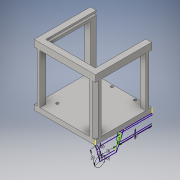
# Autodesk Inventor part: Main_Body_Wheel
Saved by Autodesk Inventor 2016 (Build 200138000, 138)
## iProperties
Created: 2018-09-17
Part Number: Main_Body_Wheel
Material: Generic
Document SubType Name: Modeling
Designer: Kyle
Density: 1 g/cm^3
Appearance: Default
Author: Kyle
Autodesk Inventor part; units mm, degrees
ref_plane "YZ Plane" through (0, 0, 0) normal (1, 0, 0) x (0, 1, 0)
ref_plane "XZ Plane" through (0, 0, 0) normal (0, 1, 0) x (-1, 0, 0)
ref_plane "XY Plane" through (0, 0, 0) normal (0, 0, 1) x (1, 0, 0)
sketch "Sketch1" plane through (0, 0, 0) normal (0, 1, 0) x (-1, 0, 0)
  line L0 (-30, 34) -> (30, 34)
  line L1 (30, 34) -> (30, -34)
  line L2 (30, -34) -> (-30, -34)
  line L3 (-30, -34) -> (-30, 34)
  line L4 (-30, 34) -> (30, -34) construction
  line L5 (30, 34) -> (-30, -34) construction
  line L6 (30, 34) -> (30, 19)
  line L7 (-30, -34) -> (-23, -34)
  line L8 (-30, -34) -> (8.5, -34)
  circle A0 centre (8.5, -31.5) radius 1.5
  circle A1 centre (-19.5, -31.5) radius 1.5
  circle A2 centre (-19.5, -31.5) radius 1.5
  circle A3 centre (24, 19) radius 1.5
  line L9 (24, 19) -> (0, 19)
  line L10 (0, 19) -> (0, 0)
  line L11 (0, 0) -> (8.5, -31.5)
  line L12 (8.5, -31.5) -> (0, -31.5)
  line L13 (-19.5, -31.5) -> (-19.5, 0)
  line L14 (-19.5, 0) -> (0, 0)
  line L15 (30, 34) -> (37, 34)
  line L16 (-37, -34) -> (37, -34)
  line L17 (37, -34) -> (37, 34)
  line L18 (37, 34) -> (-37, 34)
  line L19 (-37, 34) -> (-37, -34)
  line L20 (-37, -34) -> (37, 34) construction
  line L21 (37, -34) -> (-37, 34) construction
  dimension "d0" = 60
  dimension "d1" = 68
  dimension "d3" = 7
  dimension "d5" = 3
  dimension "d6" = 3
  dimension "d7" = 3
  dimension "d10" = 7
  dimension "d11" = 31.5
  dimension "d12" = 19.5
  dimension "d13" = 90
  dimension "d14" = 32.6267
  dimension "d15" = 8.5
  dimension "d16" = 24
  constraints: 44 end point, 5 parallel, 5 point on line, 4 centre point, 4 midpoint, 4 perpendicular, 3 horizontal, 1 coincident, 1 concentric, 1 vertical
  measures "d0" distance of L4.end L3.start
  measures "d1" distance of L5.start L4.end
  measures "d3" distance of L3.start L7.end
  measures "d5" diameter of A0
  measures "d6" diameter of A1
  measures "d7" diameter of A3
  measures "d10" distance of L5.start L20.end
  measures "d11" distance of L13.start L13.end
  measures "d12" distance of L13.end L14.end
  measures "d13" angle of L13 L14
  measures "d14" distance of L14.end L11.end
  measures "d15" distance of L11.end L12.end
  measures "d16" distance of L9.start L10.start
extrude "Extrusion1" add sketch "Sketch1" along normal blind 6
sketch "Sketch2" plane through (0, 6, 0) normal (0, 1, 0) x (1, 0, 0)
  circle A0 centre (-24, -19) radius 1.5 projected
  circle A1 centre (19.5, 31.5) radius 1.5 projected
  circle A2 centre (-8.5, 31.5) radius 1.5 projected
  line L0 (37, 34) -> (-37, 34) projected
  line L1 (-37, 34) -> (-37, -34) projected
  line L2 (-37, -34) -> (37, -34) projected
  line L3 (37, -34) -> (37, 34) projected
  line L4 (-37, 34) -> (-37, -34) projected
  line L5 (-33.5, 34) -> (-30, 34)
  line L6 (-30, 34) -> (-30, 27)
  line L7 (-30, 27) -> (-37, 27)
  line L8 (-37, 27) -> (-37, 30.5)
  line L9 (-37, 30.5) -> (-33.5, 34)
  line L10 (37, 34) -> (-37, 34) projected
  line L11 (-37, -34) -> (-30, -34)
  line L12 (-30, -34) -> (-30, -27)
  line L13 (-30, -27) -> (-37, -27)
  line L14 (-37, -27) -> (-37, -30.5)
  line L15 (-37, -34) -> (37, -34) projected
  line L16 (33.5, -34) -> (30, -34)
  line L17 (30, -34) -> (30, -27)
  line L18 (30, -27) -> (37, -27)
  line L19 (37, -27) -> (37, -30.5)
  line L20 (33.5, 34) -> (30, 34)
  line L21 (30, 34) -> (30, 27)
  line L22 (30, 27) -> (37, 27)
  line L23 (37, 27) -> (37, 30.5)
  line L24 (-30, -34) -> (-33.5, -34)
  line L25 (-33.5, -34) -> (-37, -30.5)
  line L26 (-37, -30.5) -> (-37, -27)
  line L27 (33.5, -34) -> (37, -30.5)
  line L28 (37, -34) -> (37, 34) projected
  line L29 (37, -30.5) -> (37, -27)
  line L30 (33.5, -34) -> (30, -34)
  line L31 (37, 27) -> (37, 30.5)
  line L32 (37, 30.5) -> (33.5, 34)
  line L33 (33.5, 34) -> (30, 34)
  point P0 (0, 0)
  dimension "d19" = 7
  dimension "d20" = 7
  dimension "d21" = 7
  dimension "d22" = 7
  dimension "d23" = 7
  dimension "d24" = 7
  dimension "d25" = 7
  dimension "d26" = 7
  dimension "d27" = 3.5
  constraints: 52 end point, 8 parallel, 6 perpendicular, 4 horizontal, 4 point on line, 3 collinear
  measures "d19" distance of L6.end L7.end
  measures "d20" distance of L5.end L6.end
  measures "d21" distance of L13.end L12.end
  measures "d22" distance of L12.end L11.end
  measures "d23" distance of L17.end L18.end
  measures "d24" distance of L16.end L17.end
  measures "d25" distance of L22.end L21.end
  measures "d26" distance of L21.end L20.end
  measures "d27" distance of L11.end L24.end
extrude "Extrusion2" add sketch "Sketch2" along normal blind 60 contours L32 L3 L22 L21 L0 | L6 L7 L1 L9 L0 | L3 L27 L2 L17 L18 | L13 L12 L2 L25 L1
sketch "Sketch3" plane through (0, 66, 0) normal (0, 1, 0) x (1, 0, 0)
  line L0 (37, 30.5) -> (33.5, 34) projected
  line L1 (33.5, 34) -> (30, 34) projected
  line L2 (30, 34) -> (30, 27) projected
  line L3 (30, 27) -> (37, 27) projected
  line L4 (37, 27) -> (37, 30.5) projected
  line L5 (37, -30.5) -> (37, -27) projected
  line L6 (37, -27) -> (30, -27) projected
  line L7 (30, -27) -> (30, -34) projected
  line L8 (30, -34) -> (33.5, -34) projected
  line L9 (33.5, -34) -> (37, -30.5) projected
  line L10 (-30, -34) -> (-30, -27) projected
  line L11 (-30, -27) -> (-37, -27) projected
  line L12 (-37, -27) -> (-37, -30.5) projected
  line L13 (-37, -30.5) -> (-33.5, -34) projected
  line L14 (-33.5, -34) -> (-30, -34) projected
  line L15 (-30, 27) -> (-30, 34) projected
  line L16 (-33.5, 34) -> (-37, 30.5) projected
  line L17 (-37, 30.5) -> (-37, 27) projected
  line L18 (-37, 27) -> (-30, 27) projected
  line L19 (-30, 27) -> (-30, 34) projected
  line L20 (-30, 34) -> (-33.5, 34) projected
  line L21 (-37, 34) -> (-30, 34)
  line L22 (-30, 34) -> (-30, -34)
  line L23 (-30, -34) -> (-37, -34)
  line L24 (-37, -34) -> (-37, 34)
  line L25 (30, 34) -> (30, 27) projected
  line L26 (37, -34) -> (30, -34)
  line L27 (30, -34) -> (30, 34)
  line L28 (30, 34) -> (37, 34)
  line L29 (37, 34) -> (37, -34)
  line L30 (-30, -34) -> (-30, -27) projected
  line L31 (37, -27) -> (30, -27) projected
  line L32 (-30, -34) -> (30, -34)
  line L33 (30, -34) -> (30, -27)
  line L34 (30, -27) -> (-30, -27)
  line L35 (-30, -27) -> (-30, -34)
  point P0 (0, 0)
  constraints: 24 end point, 6 parallel, 3 horizontal, 3 perpendicular, 1 point on line
extrude "Extrusion3" add sketch "Sketch3" along normal blind 8
sketch "Sketch4" plane through (37, 0, -34) normal (0, 0, -1) x (-1, 0, 0)
  line L0 (0, 66) -> (0, 74) projected
  line L1 (0, 74) -> (7, 74)
  line L2 (7, 74) -> (7, 66)
  line L3 (7, 66) -> (0, 66)
  line L4 (0, 66) -> (0, 74)
  line L5 (74, 6) -> (74, 66) projected
  line L6 (74, 66) -> (67, 66)
  line L7 (67, 66) -> (67, 74)
  line L8 (67, 74) -> (74, 74)
  line L9 (74, 74) -> (74, 66)
  line L10 (7, 66) -> (7, 69)
  line L11 (7, 66) -> (7, 74) projected
  line L12 (7, 69) -> (3.5, 69)
  line L13 (3.5, 69) -> (3.5, 72)
  line L14 (3.5, 72) -> (7, 72)
  line L15 (7, 72) -> (7, 74)
  line L16 (3.5, 72) -> (7, 72)
  line L17 (7, 72) -> (7, 69)
  line L18 (7, 69) -> (3.5, 69)
  line L19 (3.5, 69) -> (3.5, 72)
  line L20 (67, 6) -> (67, 66) projected
  line L21 (67, 66) -> (67, 69)
  line L22 (67, 66) -> (67, 74) projected
  line L23 (67, 69) -> (70.5, 69)
  line L24 (70.5, 69) -> (70.5, 72)
  line L25 (70.5, 72) -> (67, 72)
  line L26 (67, 72) -> (67, 69)
  line L27 (7, 72) -> (67, 72)
  line L28 (67, 72) -> (67, 69)
  line L29 (67, 69) -> (7, 69)
  line L30 (7, 69) -> (7, 72)
  point P0 (37, 0)
  dimension "d32" = 3
  dimension "d33" = 3
  dimension "d34" = 3
  dimension "d35" = 3.5
  dimension "d36" = 3
  constraints: 52 end point, 10 parallel, 8 perpendicular, 5 horizontal, 4 point on line, 1 vertical
  measures "d32" distance of L2.end L10.end
  measures "d33" distance of L12.end L13.end
  measures "d34" distance of L20.end L21.end
  measures "d35" distance of L25.end L24.end
  measures "d36" distance of L24.end L23.end
extrude "Extrusion4" cut sketch "Sketch4" against normal blind 64.5 contours L12 L13 L14 L2 | L2 L27 L7 L29 | L7 L25 L24 L23
sketch "Sketch5" plane through (37, 0, 34) normal (1, 0, 0) x (0, 0, -1)
  line L0 (0, 0) -> (0, 6) projected
  line L1 (0, 0) -> (5.1764, -19.3185)
  line L2 (0, 0) -> (20, 0) construction
  line L3 (5.1764, -19.3185) -> (25.1764, -19.3185)
  line L4 (5.1764, -19.3185) -> (25.1764, -19.3185) construction
  line L5 (25.1764, -19.3185) -> (34, 0)
  line L6 (29.3317, -3) -> (23.2485, -16.3185)
  line L7 (23.2485, -16.3185) -> (7.4784, -16.3185)
  line L8 (7.4784, -16.3185) -> (3.9097, -3)
  line L9 (3.9097, -3) -> (20, -3)
  line L10 (20, -3) -> (29.3317, -3)
  dimension "d39" = 20
  dimension "d40" = 75
  dimension "d41" = 20
  dimension "d42" = 0
  dimension "d43" = 3
  constraints: 20 end point, 4 horizontal, 2 equal length, 2 other
  measures "d39" distance of L0.start L1.end
  measures "d40" angle of L1 L2
  measures "d41" distance of L1.end L3.end
  measures "d42" distance between parallel lines of L3 L4
  measures "d43" distance between parallel lines of L1 L8
sketch "Sketch6" plane through (37, 0, 34) normal (1, 0, 0) x (0, 0, -1)
  line L0 (68, 0) -> (68, 6) projected
  line L1 (68, 0) -> (28, 0)
  line L2 (28, 0) -> (28, -13)
  line L3 (28, -13) -> (68, -13)
  line L4 (66, -11) -> (30, -11)
  line L5 (30, -11) -> (30, -2)
  line L6 (30, -2) -> (66, -2)
  line L7 (68, -13) -> (68, -11)
  line L8 (68, -2) -> (68, 0)
  line L9 (66, -11) -> (68, -11)
  line L10 (66, -2) -> (68, -2)
  point P0 (34, 0)
  dimension "d44" = 40
  dimension "d45" = 13
  dimension "d46" = 2
  constraints: 20 end point, 4 parallel, 3 perpendicular, 2 horizontal, 2 point on line, 2 other
  measures "d44" distance of L3.end L2.end
  measures "d45" distance of L2.end L1.end
  measures "d46" distance between parallel lines of L3 L4
body "Solid1"
